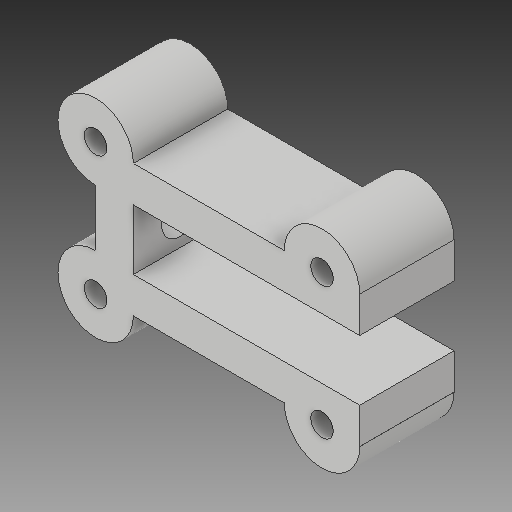
# Autodesk Inventor part: halterung_arm
Saved by Autodesk Inventor 2019 (Build 230136000, 136)
## iProperties
Created: 2017-06-08
Part Number: halterung_arm
Material: Allgemein
Document SubType Name: Modeling
Designer: eule-3
Density: 1 g/cm^3
Appearance: Vorgabe
Author: eule-3
Autodesk Inventor part; units mm, degrees
ref_plane "YZ Plane" through (0, 0, 0) normal (1, 0, 0) x (0, 1, 0)
ref_plane "XZ Plane" through (0, 0, 0) normal (0, 1, 0) x (-1, 0, 0)
ref_plane "XY Plane" through (0, 0, 0) normal (0, 0, 1) x (1, 0, 0)
sketch "Skizze1" plane through (0, 0, 0) normal (0, 0, 1) x (1, 0, 0)
  line L0 (0, 0) -> (35, 0)
  line L1 (35, 0) -> (35, 17.5)
  line L2 (35, 17.5) -> (0, 17.5)
  line L3 (0, 17.5) -> (0, 0)
  dimension "d0" = 35
  dimension "d1" = 17.5
  constraints: 8 end point, 2 parallel, 1 horizontal, 1 perpendicular
  measures "d0" distance of L1.end L2.end
  measures "d1" distance of L0.end L1.end
extrude "Extrusion1" add sketch "Skizze1" along normal blind 12.5
sketch "Skizze2" plane through (0, 0, 12.5) normal (0, 0, 1) x (1, 0, 0)
  line L0 (35, 0) -> (35, 17.5) projected
  line L1 (35, 12.75) -> (5, 12.75)
  line L2 (5, 12.75) -> (5, 4.75)
  line L3 (5, 4.75) -> (35, 4.75)
  line L4 (35, 4.75) -> (35, 12.75)
  line L5 (0, 0) -> (35, 0) projected
  dimension "d4" = 4.75
  dimension "d5" = 4.75
  dimension "d6" = 30
  constraints: 8 end point, 2 parallel, 1 horizontal, 1 perpendicular, 1 point on line
  measures "d4" distance from line of L1 L0.end
  measures "d5" distance between parallel lines of L5 L3
  measures "d6" distance of L1.start L1.end
extrude "Extrusion2" cut sketch "Skizze2" against normal blind 12.5
sketch "Skizze3" plane through (0, 0, 12.5) normal (0, 0, 1) x (1, 0, 0)
  circle A0 centre (0, 17.5) radius 5
  circle A1 centre (0, 0) radius 5
  line L0 (0, 0) -> (35, 0) projected
  circle A2 centre (30, 0) radius 5
  line L1 (35, 17.5) -> (0, 17.5) projected
  circle A3 centre (30, 17.5) radius 5
  line L2 (35, 12.75) -> (35, 17.5) projected
  dimension "d9" = 10
  dimension "d10" = 10
  dimension "d11" = 10
  dimension "d12" = 10
  constraints: 4 centre point, 2 point on line, 1 coincident
  measures "d9" diameter of A0
  measures "d10" diameter of A1
  measures "d11" diameter of A2
  measures "d12" diameter of A3
extrude "Extrusion3" cut sketch "Skizze3" against normal blind 12.5
sketch "Skizze4" plane through (0, 0, 12.5) normal (0, 0, 1) x (1, 0, 0)
  circle A0 centre (30, 17.5) radius 5
  circle A1 centre (30, 0.0223) radius 5
  circle A2 centre (0, 0) radius 5
  circle A3 centre (0, 17.5) radius 5
  line L0 (0, 12.5) -> (0, 5) projected
  line L1 (5, 4.75) -> (5, 12.75) projected
  dimension "d17" = 10
  dimension "d18" = 10
  dimension "d19" = 10
  dimension "d20" = 10
  dimension "d21" = 30
  dimension "d24" = 25
  constraints: 4 centre point
  measures "d17" diameter of A1
  measures "d18" diameter of A0
  measures "d19" diameter of A3
  measures "d20" diameter of A2
  measures "d21" distance from line of L0 A1.centre
  measures "d24" distance from line of A0.centre L1
extrude "Extrusion4" add sketch "Skizze4" against normal blind 12.5
sketch "Skizze5" plane through (0, 0, 12.5) normal (0, 0, 1) x (1, 0, 0)
  arc A0 (25, 0.0111) -> (35, 0.0111) centre (30, 0.0223) ccw projected
  point P0 (0, 0)
  point P1 (0, 0)
  point P2 (0, 17.5)
  point P3 (30, 17.5223)
  dimension "d27" = 17.5
  dimension "d28" = 17.5
  dimension "d29" = 30
  constraints: 2 coincident
  measures "d27" distance of point (0, 0) point (0, 17.5)
  measures "d28" distance of point (30, 17.522) A0.centre
  measures "d29" distance of A0.centre point (0, 0)
sketch "Skizze6" plane through (0, 0, 12.5) normal (0, 0, 1) x (1, 0, 0)
  point P0 (0, 0)
hole "Bohrung1" at (0, 0, 12.5) at (0, 17.5, 12.5) at (30, 17.5223, 12.5) at (30, 0.0223, 12.5) direction (0, 0, -1) diameter 3 end through all
sketch "Skizze8" plane through (5, 4.75, 12.5) normal (1, 0, 0) x (0, 0, -1)
  line L0 (12.5, 8) -> (12.5, 0) projected
  line L1 (12.5, 0) -> (0, 0) projected
  point P0 (12.5, -4.75)
  point P1 (6.25, 3.75)
  dimension "d37" = 6.25
  dimension "d38" = 3.75
  measures "d37" distance from line of L0 point (6.25, 3.75)
  measures "d38" distance from line of L1 point (6.25, 3.75)
hole "Bohrung2" at (5, 8.5, 6.25) direction (-1, 0, 0) diameter 5 end through all
sketch "Skizze9" plane through (5, 4.75, 12.5) normal (1, 0, 0) x (0, 0, -1)
  line L0 (12.5, 0) -> (0, 0) projected
  line L1 (0, 8) -> (12.5, 8) projected
  line L2 (0, 0) -> (12.5, 0)
  line L3 (12.5, 0) -> (12.5, 8)
  line L4 (12.5, 8) -> (0, 8)
  line L5 (0, 8) -> (0, 0)
  point P0 (12.5, -4.75)
  constraints: 8 end point, 2 parallel, 1 horizontal, 1 perpendicular
extrude "Extrusion5" cut sketch "Skizze9" along normal blind 30
